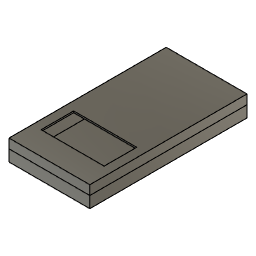
Case_completa (Autodesk Fusion 360 design; units mm, degrees)
Autodesk Fusion 360 part; units mm, degrees
sketch "Sketch2" plane through (0, 0, 0) normal (0, 0, 1) x (1, 0, 0)
  line L0 (35.634, -0.5) -> (-1.3663, -0.5)
  line L1 (-1.3663, -0.5) -> (-1.3663, 73.36)
  line L2 (-1.3663, 73.36) -> (35.634, 73.36)
  line L3 (35.634, 73.36) -> (35.634, -0.5)
  line L4 (-0.8663, 72.86) -> (-0.8663, 0) construction
  line L5 (35.634, 0) -> (-0.8663, 0) construction
  line L6 (35.134, 72.86) -> (35.134, 0) construction
  line L7 (-0.8663, 72.86) -> (35.134, 72.86) construction
  circle A0 centre (17.5, 1.8601) radius 1.45
  circle A1 centre (20.504, 70.8573) radius 1.45
  line L8 (12.32, 40.46) -> (8.32, 40.46)
  line L9 (8.32, 40.46) -> (8.32, 34.16)
  line L10 (8.32, 34.16) -> (12.32, 34.16)
  line L11 (12.32, 34.16) -> (12.32, 40.46)
  line L12 (12.02, 34.46) -> (12.02, 40.16) construction
  line L13 (12.02, 34.46) -> (8.62, 34.46) construction
  line L14 (8.62, 40.16) -> (12.02, 40.16) construction
  line L15 (8.62, 40.16) -> (8.62, 34.46) construction
  line L16 (1.8923, 25.4405) -> (32.3123, 25.4405)
  line L17 (32.3123, 25.4405) -> (32.3123, 9.7405)
  line L18 (32.3123, 9.7405) -> (1.8923, 9.7405)
  line L19 (1.8923, 9.7405) -> (1.8923, 25.4405)
  line L20 (2.3923, 24.9405) -> (31.8123, 24.9405)
  line L21 (2.3923, 10.2405) -> (2.3923, 24.9405)
  line L22 (31.8123, 24.9405) -> (31.8123, 10.2405)
  line L23 (31.8123, 10.2405) -> (2.3923, 10.2405)
  line L24 (36.634, 74.36) -> (36.634, -1.5)
  line L25 (36.634, -1.5) -> (-2.3663, -1.5)
  line L26 (-2.3663, -1.5) -> (-2.3663, 74.36)
  line L27 (-2.3663, 74.36) -> (36.634, 74.36)
  line L28 (36.134, 73.86) -> (36.134, -1)
  line L29 (36.134, -1) -> (-1.8663, -1)
  line L30 (-1.8663, -1) -> (-1.8663, 73.86)
  line L31 (-1.8663, 73.86) -> (36.134, 73.86)
  circle A2 centre (20.504, 70.8573) radius 1.2
  circle A3 centre (17.5, 1.8601) radius 1.2
  circle A4 centre (17.5, 1.8601) radius 1.7
  circle A5 centre (20.504, 70.8573) radius 1.7
  dimension "d10" = 0.5
  dimension "d11" = 0.5
  dimension "d12" = 0.5
  dimension "d13" = 0.5
  dimension "d14" = 2.9
  dimension "d15" = 2.9
  dimension "d20" = 0.3
  dimension "d21" = 0.3
  dimension "d22" = 0.3
  dimension "d23" = 0.3
  dimension "d24" = 0.5
  dimension "d25" = 0.5
  dimension "d26" = 0.5
  dimension "d27" = 0.5
  dimension "d30" = -1
  dimension "d35" = -0.5
  dimension "d39" = -0.25
  dimension "d40" = -0.25
  dimension "d57" = 0.25
  dimension "d58" = 0.25
  constraint horizontal L0
  constraint vertical L1
  constraint horizontal L2
  constraint vertical L3
  constraint perpendicular L0 L4
  constraint perpendicular L4 L5
  constraint coincident L5.start L3
  constraint coincident L5 L6.end
  constraint perpendicular L5 L6
  constraint perpendicular L6 L7
  constraint horizontal L8
  constraint vertical L9
  constraint horizontal L10
  constraint vertical L11
  constraint perpendicular L8 L12
  constraint perpendicular L9 L13
  constraint perpendicular L11 L14
  constraint perpendicular L10 L15
  constraint horizontal L16
  constraint vertical L17
  constraint horizontal L18
  constraint vertical L19
  measures "d10" distance of L1 L4
  measures "d11" distance of L0 L5
  measures "d12" distance of L2 L7
  measures "d13" distance of L3 L6
  measures "d14" diameter of A0
  measures "d15" diameter of A1
  measures "d20" distance of L8 L14
  measures "d21" distance of L9 L15
  measures "d22" distance of L10 L13
  measures "d23" distance of L11 L12
  measures "d24" distance of L16 L20
  measures "d25" distance of L19 L21
  measures "d26" distance of L17 L22
  measures "d27" distance of L18 L23
extrude "Extrude2" add sketch "Sketch2" along normal blind 6 contours L24 L25 L26 L27 | L28 L29 L30 L31 makes body 1
extrude "Extrude3" add sketch "Sketch2" along normal blind 0.75 separate body contours L0 L1 L2 L3 | A0 | A1 | L16 L17 L18 L19 | L20 L21 L22 L23 | A2 | A3 | A4 | A5 makes body 2
combine "Combine1" operation add target body 2 tool bodies 1
extrude "Extrude4" cut sketch "Sketch2" against normal blind 0.5 from surface at 6 contours L24 L25 L26 L27 bodies 2
extrude "Extrude5" cut sketch "Sketch2" along normal blind 1 contours A2 | A3 bodies 2
extrude "Extrude6" add sketch "Sketch2" against normal blind 0.75 from surface at 10 separate body contours L0 L1 L2 L3 | A0 | A1 | L8 L9 L10 L11 | L24 L25 L26 L27 | L28 L29 L30 L31 | A2 | A3 | A4 | A5 makes body 3
extrude "Extrude7" add sketch "Sketch2" against normal blind 3.25 from surface at 9.25 separate body contours L24 L25 L26 L27 | L28 L29 L30 L31 makes body 4
combine "Combine2" operation add target body 3 tool bodies 4
extrude "Extrude8" add sketch "Sketch2" against normal blind 0.5 from surface at 6 separate body contours L24 L25 L26 L27 makes body 5
combine "Combine3" operation add target body 3 tool bodies 5
extrude "Extrude9" add sketch "Sketch2" against normal blind 3.75 from surface at 9.25 contours A0 | A1 bodies 3
extrude "Extrude10" add sketch "Sketch2" along normal blind 5.5 separate body contours A0 | A1 makes body 6 at (18.9482, 1.7878, 3.6667) makes body 7 at (21.9522, 70.7851, 3.6667)
combine "Combine4" operation add target body 7 tool bodies 6 2
extrude "Extrude11" add sketch "Sketch2" along normal blind 3 contours A4 | A5 bodies 7
copy_body "Body->Comp1" bodies 3 removing the originals makes body 8 in component "Tampa"
copy_body "Body->Comp2" bodies 7 removing the originals makes body 9 in component "Base"
component "Tampa" placed x (1, 0, 0) y (0, 1, 0) z (0, 0, 1) at (0, 0, 0)
component "Base" placed x (1, 0, 0) y (0, 1, 0) z (0, 0, 1) at (0, 0, 0)
named bodies: "Tampa", "Base"
